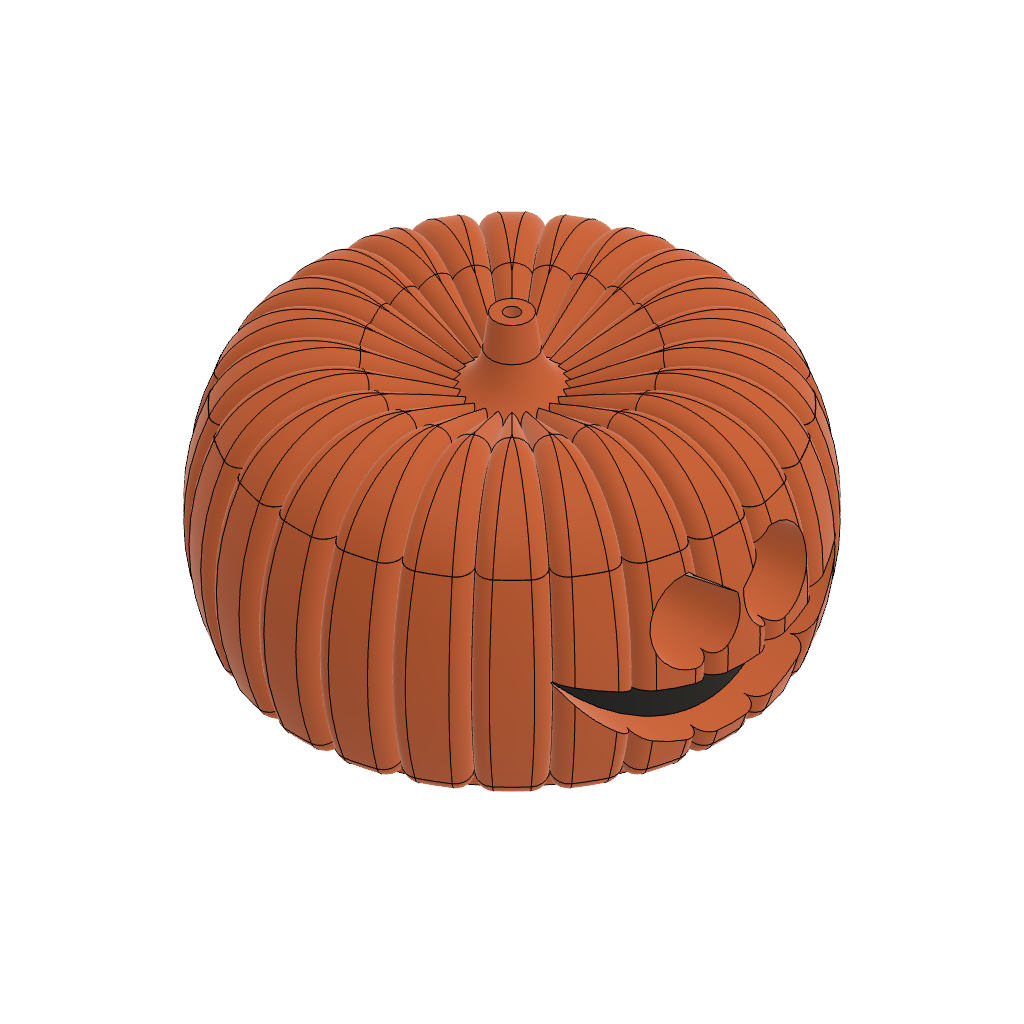
TinyEngineerHalloween (Autodesk Fusion 360 design; units mm, degrees)
part number: 2026-08-31-21-58-55-159
part number: 2026-08-31-22-02-30-810
part number: 2026-08-31-23-17-40-355
part number: 2026-08-31-23-21-15-111
part number: 2026-09-02-10-24-00-688
part number: 2026-09-25-21-20-39-307
part number: 2026-09-26-07-19-26-809
Autodesk Fusion 360 part; units mm, degrees
(part 1 of 2)
sketch "servo_profile" plane through (0, 0, 0) normal (0, 0, 1) x (1, 0, 0) in component "Servo"
  line L0 (-16.9, -13.6) -> (-16.9, -30.6) construction
  line L1 (-16.9, -30.6) -> (5.8, -30.6) construction
  line L2 (5.8, -30.6) -> (5.8, -13.6) construction
  line L3 (5.8, -13.6) -> (10.6, -13.6) construction
  line L4 (10.6, -13.6) -> (10.6, -11.2) construction
  line L5 (10.6, -11.2) -> (5.8, -11.2) construction
  line L6 (5.8, -3.3) -> (-9.1, -3.3) construction
  line L7 (-9.1, -3.3) -> (-9.1, -6.8) construction
  line L8 (-9.1, -6.8) -> (-16.9, -6.8) construction
  line L9 (-16.9, -6.8) -> (-16.9, -11.2) construction
  line L10 (-16.9, -11.2) -> (-21.7, -11.2) construction
  line L11 (-21.7, -11.2) -> (-21.7, -13.6) construction
  line L12 (-21.7, -13.6) -> (-16.9, -13.6) construction
  line L13 (0, -3.3) -> (0, 0) construction
  line L14 (5.8, -3.3) -> (5.8, -11.2) construction
  line L15 (-17.2, -10.9) -> (-22, -10.9)
  line L16 (-22, -10.9) -> (-22, -13.9)
  line L17 (-22, -13.9) -> (-17.2, -13.9)
  line L18 (-17.2, -13.9) -> (-17.2, -30.9)
  line L19 (-17.2, -30.9) -> (6.1, -30.9)
  line L20 (6.1, -30.9) -> (6.1, -13.9)
  line L21 (6.1, -13.9) -> (10.9, -13.9)
  line L22 (10.9, -13.9) -> (10.9, -10.9)
  line L23 (10.9, -10.9) -> (6.1, -10.9)
  line L24 (6.1, -3) -> (6.1, -10.9)
  line L25 (6.1, -3) -> (-9.4, -3)
  line L26 (-9.4, -3) -> (-9.4, -6.5)
  line L27 (-9.4, -6.5) -> (-17.2, -6.5)
  line L28 (-17.2, -6.5) -> (-17.2, -10.9)
  line L29 (-9.1, -3.3) -> (-16.9, -3.3) construction
  line L30 (-16.9, -3.3) -> (-16.9, -6.8) construction
  dimension "d2" = 22.7
  dimension "d6" = 17
  dimension "d7" = 2.4
  dimension "d8" = 4.8
  dimension "d13" = 4.4
  dimension "d17" = 5.8
  dimension "d20" = 3.3
  dimension "d40" = 0.3
  dimension "d115" = 3.5
  dimension "d116" = 7.8
  constraint vertical L0
  constraint perpendicular L0 L1
  constraint perpendicular L1 L2
  constraint perpendicular L0 L3
  constraint perpendicular L3 L4
  constraint perpendicular L4 L5
  constraint perpendicular L6 L7
  constraint perpendicular L7 L8
  constraint perpendicular L8 L9
  constraint perpendicular L9 L10
  constraint perpendicular L10 L11
  constraint perpendicular L0 L12
  constraint equal L0 L2
  constraint equal L4 L11
  constraint collinear L0 L9
  constraint equal L3 L12
  constraint coincident L6 L13.start
  constraint perpendicular L6 L13
  constraint coincident L13.end origin
  constraint perpendicular L5 L14
  constraint collinear L2 L14
  constraint coincident L6.start L14.start
  constraint perpendicular L26 L29
  constraint perpendicular L29 L30
  measures "d2" distance of L0.end L1.end
  measures "d6" distance of L0.start L0.end
  measures "d7" distance of L10.end L11.end
  measures "d8" distance of L2.end L3.end
  measures "d13" distance of L8.end L9.end
  measures "d17" distance of L13 L14
  measures "d20" distance of L13.start L13.end
  measures "d115" distance of L8.end L29.end
  measures "d116" distance of L6.end L29.end
extrude "Extrude1" add sketch "servo_profile" along normal mid plane 12.8 makes body 1 in component "Servo"
sketch "shaft" plane through (0, -3, 0) normal (0, 1, 0) x (-1, 0, 0) in component "Servo"
  line L0 (9, -5.75) -> (9, 5.75)
  line L1 (9, 5.75) -> (-3, 5.75)
  line L2 (-3, 5.75) -> (-3, -5.75)
  line L3 (-3, -5.75) -> (9, -5.75)
  circle A0 centre (0, 0) radius 2.7
  line L4 (9.4, -6.4) -> (9.4, 6.4)
  line L5 (9.4, 6.4) -> (-6.1, 6.4)
  line L6 (-6.1, 6.4) -> (-6.1, -6.4)
  line L7 (-6.1, -6.4) -> (9.4, -6.4)
  dimension "d25" = 5.4
  constraint coincident A0.centre origin
  measures "d25" diameter of A0
extrude "Extrude2" add sketch "shaft" along normal blind 3.6 contours A0 bodies 1 in component "Servo"
sketch "mount" plane through (0, -3, 0) normal (0, 1, 0) x (-1, 0, 0) in component "Servo"
  circle A0 centre (-8.27, 0) radius 1.4
  circle A1 centre (19.37, 0) radius 1.4
  line L0 (19.37, 0) -> (-8.27, 0) construction
  line L1 (0, 0) -> (-5.8, 0) construction
  line L2 (-5.8, 0) -> (-10.6, 0) construction
  line L3 (-10.6, 0) -> (-10.6, -6.1) construction
  line L4 (-10.6, -6.1) -> (-8.27, -6.1) construction
  line L5 (-8.27, -6.1) -> (-8.27, 0) construction
  dimension "d31" = 2.8
  dimension "d32" = 5.8
  dimension "d33" = 4.8
  dimension "d34" = 6.1
  dimension "d35" = 2.33
  dimension "d36" = 6.1
  dimension "d37" = 19.37
  constraint coincident A1.centre L0.start
  constraint coincident A0.centre L0.end
  constraint horizontal L0
  constraint equal A0 A1
  constraint coincident L1.start origin
  constraint horizontal L1
  constraint parallel L1 L2
  constraint perpendicular L2 L3
  constraint perpendicular L3 L4
  constraint vertical L5
  measures "d31" diameter of A0
  measures "d32" distance of L1.start L1.end
  measures "d33" distance of L1.end L2.end
  measures "d34" distance of L2.end L3.end
  measures "d35" distance of L3.end L4.end
  measures "d36" distance of A0.centre L4.end
  measures "d37" distance of L1.start A1.centre
extrude "Extrude3" cut sketch "mount" against normal through all bodies 1 in component "Servo"
sketch "Sketch1" plane through (0, 0, 0) normal (0, 0, 1) x (1, 0, 0) in component "OLED"
  line L0 (-4.7, -18.25) -> (0, -18.25)
  line L1 (0, -18.25) -> (0, 18.25)
  line L2 (0, 18.25) -> (-8.7, 18.25)
  line L3 (-8.7, 18.25) -> (-8.7, 10.25)
  line L4 (-8.7, 10.25) -> (-4.7, 10.25)
  line L5 (-4.7, 10.25) -> (-4.7, -18.25)
  dimension "d195" = 36.5
  dimension "d196" = 4.7
  dimension "d197" = 8.7
  dimension "d202" = 8
  constraint horizontal L0
  constraint perpendicular L0 L1
  constraint perpendicular L1 L2
  constraint perpendicular L2 L3
  constraint perpendicular L3 L4
  constraint perpendicular L4 L5
  constraint midpoint origin L1
  measures "d195" distance of L0.end L1.end
  measures "d196" distance of L0.start L0.end
  measures "d197" distance of L1.end L2.end
  measures "d202" distance of L2.end L3.end
extrude "Extrude1'" add sketch "Sketch1" along normal blind 12.5 separate body makes body 2 in component "OLED"
sketch "servo_case" plane through (0, 0, -6.4) normal (0, 0, -1) x (1, 0, 0) in component "Head"
  line L0 (-9.4, 3) -> (6.1, 3)
  line L1 (6.1, 3) -> (6.1, 10.9)
  line L2 (6.1, 10.9) -> (10.9, 10.9)
  line L3 (10.9, 13.9) -> (6.1, 13.9)
  line L4 (6.1, 13.9) -> (6.1, 30.9)
  line L5 (6.1, 30.9) -> (-17.2, 30.9)
  line L6 (-17.2, 30.9) -> (-17.2, 13.9)
  line L7 (-17.2, 13.9) -> (-22, 13.9)
  line L8 (-22, 10.9) -> (-17.2, 10.9)
  line L9 (-17.2, 10.9) -> (-17.2, 6.5)
  line L10 (-17.2, 6.5) -> (-9.4, 6.5)
  line L11 (-9.4, 6.5) -> (-9.4, 3)
  line L12 (12.1, 3) -> (-23.5, 3)
  line L13 (-23.5, 3) -> (-23.5, 35.9) construction
  line L14 (-23.5, 35.9) -> (12.1, 35.9)
  line L15 (12.1, 35.9) -> (12.1, 3)
  line L16 (6.1, 3) -> (6.1, 10.9)
  line L17 (6.1, 10.9) -> (10.9, 10.9)
  line L18 (10.9, 10.9) -> (10.9, 13.9)
  line L19 (10.9, 13.9) -> (6.1, 13.9)
  line L20 (6.1, 13.9) -> (6.1, 30.9)
  line L21 (6.1, 30.9) -> (-17.2, 30.9)
  line L22 (-17.2, 30.9) -> (-17.2, 13.9)
  line L23 (-17.2, 13.9) -> (-22, 13.9)
  line L24 (-22, 13.9) -> (-22, 10.9)
  line L25 (-22, 10.9) -> (-17.2, 10.9)
  line L26 (-17.2, 10.9) -> (-17.2, 6.5)
  line L27 (-17.2, 6.5) -> (-9.4, 6.5)
  line L28 (-9.4, 6.5) -> (-9.4, 3)
  line L29 (12.1, 35.9) -> (12.1, 24.9)
  line L30 (12.1, 24.9) -> (11.6, 24.9) construction
  line L31 (8.6, 34.4) -> (8.6, 32.9) construction
  line L32 (7.1, 32.9) -> (6.1, 32.9)
  line L33 (4.1, 32.9) -> (4.1, 30.9) construction
  line L34 (11.6, 24.9) -> (11.6, 35.9)
  line L35 (11.6, 24.9) -> (6.1, 24.9)
  line L36 (-5.55, 30.9) -> (-5.55, 19) construction
  circle A0 centre (-5.55, 19) radius 9.85
  line L37 (10.9, 10.9) -> (10.9, 13.9)
  line L38 (-22, 13.9) -> (-22, 10.9)
  line L39 (8.6, 34.4) -> (7.1, 34.4) construction
  line L40 (8.6, 35.9) -> (8.6, 34.4) construction
  arc A1 (7.1, 32.9) -> (7.1, 35.9) centre (7.1, 34.4) ccw
  line L41 (8.6, 32.9) -> (7.1, 32.9) construction
  arc A2 (6.1, 32.9) -> (4.1, 30.9) centre (6.1, 30.9) ccw
  line L42 (6.1, 32.9) -> (4.1, 32.9) construction
  line L43 (-53.5, 3) -> (-53.5, 35.9) construction
  line L44 (-53.5, 3) -> (-23.5, 3) construction
  line L45 (12.1, 19.45) -> (0.3, 19.45) construction
  circle A3 centre (0.3, 19.45) radius 28.9317
  line L46 (12.1, 3) -> (12.1, -6.966)
  line L47 (12.1, 35.9) -> (12.1, 45.866)
  line L48 (-21.2, 35.9) -> (-21.2, 38.8096)
  line L49 (-21.2, 3) -> (-21.2, 0.0904)
  line L50 (-16.6452, 35.9) -> (-16.6452, 42.9)
  line L51 (-16.6452, 3) -> (-16.6452, -4)
  line L52 (-17.2, 16.9) -> (-28.5191, 16.9)
  line L53 (-17.2, 27.9) -> (-27.3702, 27.9)
  point P0 (8.6, 34.4)
  dimension "d42" = 5
  dimension "d61" = 8
  dimension "d62" = 2
  dimension "d71" = 0.5
  dimension "d72" = 3
  dimension "d74" = 2
  dimension "d82" = 11.9
  dimension "d83" = 19.7
  dimension "d89" = 6.3
  dimension "d90" = 6
  dimension "head_width" = 32.9
  dimension "d267" = 30
  dimension "d1884" = 5.8
  dimension "d1981" = 2.3
  dimension "d1982" = 7
  dimension "d1999" = 3
  dimension "d2000" = 3
  dimension "d2054" = 57.8634
  constraint horizontal L12
  constraint vertical L13
  constraint horizontal L14
  constraint vertical L15
  constraint collinear L0 L12
  constraint coincident L0.end L1.start
  constraint coincident L1.end L2.start
  constraint coincident L2.end L17.end
  constraint coincident L3.start L18.end
  constraint coincident L3.end L4.start
  constraint coincident L4.end L5.start
  constraint coincident L5.end L6.start
  constraint coincident L6.end L7.start
  constraint coincident L7.end L23.end
  constraint coincident L8.start L24.end
  constraint coincident L8.end L9.start
  constraint coincident L9.end L10.start
  constraint coincident L10.end L11.start
  constraint coincident L0.start L11.end
  constraint coincident L15 L29.end
  constraint coincident L20 L35.end
  constraint perpendicular L20 L30
  constraint coincident L14 L40.start
  constraint perpendicular L14 L31
  constraint perpendicular L31 L32
  constraint coincident L21 L33.end
  constraint perpendicular L21 L33
  constraint coincident L14 L34.end
  constraint perpendicular L14 L34
  constraint perpendicular L20 L35
  constraint midpoint L21 L36.start
  constraint perpendicular L21 L36
  constraint coincident L36.end A0.centre
  constraint perpendicular L31 L39
  constraint perpendicular L14 L40
  constraint coincident P0 L31.start
  constraint equal L39 L40
  constraint equal L31 L40
  constraint coincident L14 A1.end
  constraint coincident L39.end A1.centre
  constraint perpendicular L31 L41
  constraint perpendicular L31 L42
  constraint tangent L14 A1
  constraint perpendicular L21 L43
  constraint perpendicular L43 L44
  constraint midpoint L15 L45.start
  constraint perpendicular L20 L45
  constraint coincident L45.end A3.centre
  constraint coincident L12.end A3
  constraint coincident A3 L46.end
  constraint perpendicular L12 L46
  constraint coincident A3 L47.end
  constraint perpendicular L14 L47
  constraint coincident L14 L48.start
  constraint coincident A3 L48.end
  constraint perpendicular L14 L48
  constraint coincident L12 L49.start
  constraint coincident A3 L49.end
  constraint perpendicular L12 L49
  constraint collinear L48 L49
  constraint coincident L14 L50.start
  constraint coincident A3 L50.end
  constraint perpendicular L14 L50
  constraint coincident L12 L51.start
  constraint coincident A3 L51.end
  constraint perpendicular L12 L51
  constraint collinear L50 L51
  constraint coincident L22 L52.start
  constraint coincident A3 L52.end
  constraint perpendicular L13 L52
  constraint coincident L22 L53.start
  constraint coincident A3 L53.end
  constraint perpendicular L13 L53
  measures "d42" distance of L5 L14
  measures "d61" distance of L30 L32
  measures "d62" distance of L33.start L33.end
  measures "d71" distance of L29 L34
  measures "d72" distance of L40.start L34
  measures "d74" distance of L4.end L33
  measures "d82" distance of L36.start L36.end
  measures "d83" diameter of A0
  measures "d89" distance of L13 L26
  measures "d90" distance of L15 L16
  measures "head_width" distance of L43.start L43.end
  measures "d267" distance of L12.end L43.start
  measures "d1884" horizontal distance of L0.end L45.end
  measures "d1981" distance of L13.end L48.start
  measures "d1982" distance of L50.start L50.end
  measures "d1999" distance of L5.end L53.start
  measures "d2000" distance of L23 L52
  measures "d2054" diameter of A3
extrude "Extrude1''" add sketch "servo_case" along normal blind 1.8 separate body contours L0 L1 L2 L3 L4 L5 L6 L7 L8 L9 L10 L11 L12 L16 L17 L18 L19 L20 L21 L22 L23 L24 L25 L26 L27 L28 L37 L38 | L6 L7 L8 L9 L10 L11 L12 L22 L23 L24 L25 L26 L27 L28 L38 A3 L52 | L1 L2 L3 L4 L12 L14 L15 L16 L17 L18 L19 L20 L29 L34 L35 L37 | L12 A3 L49 L51 | L15 L29 A3 L46 L47 | L6 L22 A3 L52 L53 | L4 L5 L14 L20 L21 L32 L34 L35 A1 A2 | L5 L6 L14 L21 L22 L32 A1 A2 A3 L53 | L14 A3 L48 L50 makes body 3 in component "Head"
fillet "Fillet8" radius 5 2 edges at (-16.6452, -35.9, -7.3) (-16.6452, -3, -7.3) on bodies 3 in component "Head"
fillet "Fillet8" radius 1 2 edges at (-16.6452, -42.9, -7.3) (-16.6452, 4, -7.3) on bodies 3 in component "Head"
extrude "Extrude2'" add sketch "servo_case" against normal blind 12.8 contours L6 L7 L8 L9 L10 L11 L12 L22 L23 L24 L25 L26 L27 L28 L38 A3 L52 | L1 L2 L3 L4 L12 L14 L15 L16 L17 L18 L19 L20 L29 L34 L35 L37 | L6 L22 A3 L52 L53 | L5 L6 L14 L21 L22 L32 A1 A2 A3 L53 bodies 3 in component "Head"
extrude "Extrude19" add 1 faces at (17.8106, -19.45, -6.4) along direction (0, 0, 1) up to surface (12.8 mm away) separate body on bodies 3 makes body 4 in component "Head"
fillet "Fillet12" radius 2 4 edges at (12.1, 6.966, -7.3) (12.1, -45.866, -7.3) (12.1, 6.966, 0) (12.1, -45.866, 0) on bodies 3 4 in component "Head"
shell "Shell1" thickness 1.5 removed faces 1 at (17.8106, -19.45, 6.4) on bodies 4 in component "Head"
combine "Combine1" operation add target body 3 tool bodies 4 in component "Head"
extrude "Extrude14" add sketch "servo_case" against normal blind 1 contours L4 L5 L14 L20 L21 L32 L34 L35 A1 A2 bodies 3 in component "Head"
fillet "Fillet6" radius 2 1 edges at (11.6, -24.9, 0) on bodies 3 in component "Head"
sketch "axis_mount" plane through (0, -35.9, 0) normal (0, -1, 0) x (1, 0, 0) in component "Head"
  line L0 (12.1, 6.4) -> (11.6, 6.4)
  circle A0 centre (0, 0) radius 2.7 construction
  circle A1 centre (0, 0) radius 1.2
  line L1 (11.6, 6.4) -> (11.6, -5.4)
  line L2 (11.6, -5.4) -> (7.1, -5.4)
  line L3 (-23.5, 6.4) -> (-23.5, -8.2)
  line L4 (-23.5, -8.2) -> (-21.2, -8.2)
  line L5 (7.1, -5.4) -> (7.1, 6.4)
  line L6 (7.1, 6.4) -> (-23.5, 6.4)
  line L7 (-21.2, -8.2) -> (-21.2, -6.4)
  line L8 (-21.2, -6.4) -> (-11.6452, -6.4)
  line L9 (-11.6452, -6.4) -> (-11.6452, -8.2)
  line L10 (-11.6452, -8.2) -> (12.1, -8.2)
  line L11 (12.1, -8.2) -> (12.1, 6.4)
  dimension "d106" = 2.4
  constraint concentric A0 A1
  measures "d106" diameter of A1
extrude "Extrude6" cut sketch "axis_mount" against normal up to surface (5 mm away) contours A1 bodies 3 in component "Head"
ref_plane "WorkPlane2" through (-28.6317, -19.45, -3.5582) normal (-1, 0, 0) x (0, -1, 0) in component "Head"
sketch "mount_hole" plane through (-28.6317, 0, 0) normal (-1, 0, 0) x (0, -1, 0) in component "Head"
  line L0 (3, -8.2) -> (35.9, -8.2)
  line L1 (19.45, -8.2) -> (19.45, -4.55)
  circle A0 centre (19.45, -4.55) radius 1.05
  dimension "d2018" = 3.65
  dimension "d2019" = 2.1
  constraint midpoint L0 L1.start
  constraint perpendicular L0 L1
  constraint coincident L1.end A0.centre
  measures "d2018" distance of L1.start L1.end
  measures "d2019" diameter of A0
extrude "Extrude15" cut sketch "mount_hole" against normal up to surface (9.9317 mm away) bodies 3 in component "Head"
extrude "Extrude16" cut sketch "servo_case" along normal up to surface (8.6 mm away) from surface at -12.8 contours L6 L22 A3 L52 L53 bodies 3 in component "Head"
fillet "Fillet11" radius 3 2 edges at (-28.5191, -16.9, 2.1) (-27.3702, -27.9, 2.1) on bodies 3 in component "Head"
sketch "Sketch8" plane through (0, -3, 0) normal (0, 1, 0) x (-1, 0, 0) in component "Head"
  line L0 (11.6452, -8.2) -> (11.6452, -6.4)
  line L1 (11.6452, -6.4) -> (21.2, -6.4)
  line L2 (21.2, -6.4) -> (21.2, -8.2)
  line L3 (21.2, -8.2) -> (23.5, -8.2)
  line L4 (23.5, -8.2) -> (23.5, 6.4)
  line L5 (23.5, 6.4) -> (9.4, 6.4)
  line L6 (9.4, 6.4) -> (9.4, -6.4)
  line L7 (9.4, -6.4) -> (-6.1, -6.4)
  line L8 (-6.1, -6.4) -> (-6.1, 6.4)
  line L9 (-6.1, 6.4) -> (-12.1, 6.4)
  line L10 (-12.1, 6.4) -> (-12.1, -8.2)
  line L11 (-12.1, -8.2) -> (11.6452, -8.2)
  circle A0 centre (-8.27, 0) radius 1.4 construction
  circle A1 centre (19.37, 0) radius 1.4 construction
  circle A2 centre (-8.27, 0) radius 1.05
  circle A3 centre (19.37, 0) radius 1.05
  circle A4 centre (-8.27, 0) radius 2
  circle A5 centre (19.37, 0) radius 2
  dimension "d2027" = 2.1
  dimension "d2028" = 4
  constraint concentric A0 A2
  constraint concentric A1 A3
  constraint equal A2 A3
  constraint concentric A2 A4
  constraint concentric A3 A5
  constraint equal A4 A5
  measures "d2027" diameter of A2
  measures "d2028" diameter of A5
extrude "Extrude17" cut sketch "Sketch8" against normal up to surface (27.9 mm away) contours A2 | A3 bodies 3 in component "Head"
extrude "Extrude18" cut sketch "Sketch8" against normal blind 2 contours A4 | A5 bodies 3 in component "Head"
sketch "base" plane through (0, 0, -8.2) normal (0, 0, -1) x (1, 0, 0) in component "Cover"
  circle A0 centre (-5.55, 19) radius 9.85
  arc A1 (-18.2875, 41.6209) -> (-21.2, 38.8096) centre (0.3, 19.45) ccw
  line L0 (-23.5, 3) -> (-21.2, 3)
  line L1 (12.1, 3) -> (12.1, -3.6774)
  arc A2 (15.1248, -5.3949) -> (15.1248, 44.2949) centre (0.3, 19.45) ccw
  line L2 (12.1, 42.5774) -> (12.1, 35.9)
  line L3 (12.1, 35.9) -> (-11.6452, 35.9)
  line L4 (-19.793, 40.2662) -> (0.3, 19.45) construction
  line L5 (6.1, 10.9) -> (6.1, 3)
  circle A3 centre (0.3, 19.45) radius 29.2317
  circle A4 centre (0.3, 19.45) radius 29.6317
  line L6 (-19.793, 40.2662) -> (-20.0013, 40.4821) construction
  line L7 (-20.0013, 40.4821) -> (-20.2791, 40.7699) construction
  line L8 (-21.6568, 38.7474) -> (-21.6568, 36.2)
  line L9 (-21.6568, 36.2) -> (-23.6568, 36.2)
  line L10 (-21.8636, 38.5096) -> (-21.6568, 38.5096)
  line L11 (-21.6568, 0.1526) -> (-21.6568, 38.5096)
  arc A5 (-16.6451, 40.8621) -> (-11.6452, 35.9) centre (-11.6452, 40.9) ccw
  line L12 (-21.2, 38.8096) -> (-21.2, 35.9)
  line L13 (-21.2, 35.9) -> (-23.5, 35.9)
  line L14 (-21.2, 3) -> (-21.2, 0.0904)
  arc A6 (-21.2, 0.0904) -> (-18.2875, -2.7209) centre (0.3, 19.45) ccw
  arc A7 (-11.6452, 3) -> (-16.6451, -1.9621) centre (-11.6452, -2) ccw
  line L15 (-11.6452, 3) -> (12.1, 3)
  line L16 (-21.6568, 2.7) -> (-23.6568, 2.7)
  arc A8 (-18.2875, -2.7209) -> (-16.6451, -1.9621) centre (-17.645, -1.9546) ccw
  arc A9 (-16.6451, 40.8621) -> (-18.2875, 41.6209) centre (-17.645, 40.8546) ccw
  arc A10 (15.1248, 44.2949) -> (12.1, 42.5774) centre (14.1, 42.5774) ccw
  arc A11 (12.1, -3.6774) -> (15.1248, -5.3949) centre (14.1, -3.6774) ccw
  arc A12 (-23.5, 35.9) -> (-23.5, 3) centre (0.3, 19.45) ccw
  dimension "d1885" = 5.8
  dimension "d1886" = 0.3
  dimension "d1887" = 0.4
  dimension "d1890" = 0.3
  dimension "d1891" = 0.3
  dimension "d1892" = 2
  dimension "d1985" = 2
  constraint midpoint A1 L4.start
  constraint perpendicular A1 L4
  constraint concentric A1 A3
  constraint coincident A1.centre A2.centre
  constraint coincident A3 L6.end
  constraint perpendicular A3 L6
  constraint coincident A4 L7.end
  constraint perpendicular A4 L7
  constraint coincident A3 L8.start
  constraint perpendicular L3 L8
  constraint coincident A3 L9.end
  constraint perpendicular L8 L9
  constraint coincident A3 L10.start
  constraint parallel L3 L10
  constraint coincident A3 L11.start
  constraint perpendicular L10 L11
  constraint collinear L8 L11
  constraint coincident L11 L16.start
  constraint coincident A3 L16.end
  constraint perpendicular L11 L16
  measures "d1885" horizontal distance of A1.centre L5.end
  measures "d1886" distance of L4.start L6.end
  measures "d1887" distance of L6.end L7.end
  measures "d1890" vertical distance of L3.end L8.end
  measures "d1891" vertical distance of A1.end L10.end
  measures "d1892" distance of L8.end L9.end
  measures "d1985" distance of L16.start L16.end
extrude "Extrude1'''" add sketch "base" against normal up to surface (14.6 mm away) separate body contours A3 L8 L9 L10 L11 | A3 L11 L16 | A3 L8 L10 | A4 makes body 5 in component "Cover"
sketch "oled_profile" plane through (0, 0, 6.4) normal (0, 0, 1) x (-1, 0, 0) in component "Cover"
  arc A0 (21.6568, 38.7474) -> (21.6568, 0.1526) centre (-0.3, 19.45) ccw
  line L0 (21.6568, 38.7474) -> (21.6568, 36.2)
  circle A1 centre (-0.3, 19.45) radius 29.6317
  line L1 (-22.8918, 38) -> (-17.5918, 38)
  line L2 (-17.5918, 9.5) -> (-13.5918, 9.5)
  line L3 (-17.5918, 9.5) -> (-17.5918, 38)
  line L4 (-13.5918, 9.5) -> (-13.5918, 0.9)
  line L5 (-13.5918, 0.9) -> (-22.8918, 0.9)
  line L6 (-22.8918, 0.9) -> (-22.8918, 38)
  line L7 (-19.9918, 0.9) -> (-19.9918, -2.1538)
  line L8 (-13.5918, 0.9) -> (-13.5918, -4.585)
  line L9 (-13.5918, -4.585) -> (-13.5918, -6.585) construction
  line L10 (-13.5918, -4.585) -> (-12.0918, -4.585)
  line L11 (-12.0918, -4.585) -> (-12.0918, 46.1978)
  arc A2 (-12.0918, 46.1978) -> (-19.9918, -2.1538) centre (-0.3, 19.45) ccw
  line L12 (21.6568, 36.2) -> (23.6568, 36.2)
  line L13 (21.6568, 2.7) -> (21.6568, 0.1526)
  arc A3 (23.6568, 2.7) -> (23.6568, 36.2) centre (-0.3, 19.45) ccw
  line L14 (23.6568, 2.7) -> (21.6568, 2.7)
  line L15 (-17.5918, 9.5) -> (-22.8918, 9.5)
  line L16 (-17.5918, 33) -> (-22.8918, 33)
  line L17 (21.6568, 36.2) -> (21.6568, 2.7)
  dimension "d1895" = 37.1
  dimension "d1896" = 5.3
  dimension "d1897" = 8.6
  dimension "d1898" = 9.3
  dimension "d1962" = 2.9
  dimension "d1963" = 2
  dimension "d1964" = 1.5
  dimension "d1997" = 5
  constraint horizontal L1
  constraint parallel L1 L2
  constraint perpendicular L1 L3
  constraint perpendicular L2 L4
  constraint perpendicular L4 L5
  constraint perpendicular L5 L6
  constraint coincident A0 L1.start
  constraint coincident A0 L5.end
  constraint coincident L5 L7.start
  constraint coincident A0 L7.end
  constraint perpendicular L5 L7
  constraint perpendicular L5 L8
  constraint coincident A0 L9.end
  constraint parallel L8 L9
  constraint perpendicular L9 L10
  constraint coincident A0 L11.end
  constraint vertical L11
  constraint coincident A0.centre A1.centre
  constraint coincident L6 L15.end
  constraint perpendicular L6 L15
  constraint coincident L3 L16.start
  constraint coincident L6 L16.end
  constraint perpendicular L6 L16
  constraint coincident L0.end L12.start
  constraint coincident L13.start L14.end
  measures "d1895" distance of L1.start L5.end
  measures "d1896" distance of L1.start L1.end
  measures "d1897" distance of L2.end L4.end
  measures "d1898" distance of L4.end L5.end
  measures "d1962" horizontal distance of L5.end L7.end
  measures "d1963" distance of L8.end L9.end
  measures "d1964" distance of L8.end L10.end
  measures "d1997" distance of L1.end L16.start
extrude "Extrude2''" add sketch "oled_profile" along normal blind 13.1 contours A0 L1 L2 L3 L4 L8 L10 L11 A2 | L12 A3 L14 L17 | A0 L6 A2 | A0 L5 L7 A2 | A1 bodies 5 in component "Cover"
sketch "roof" plane through (0, 0, 19.5) normal (0, 0, 1) x (-1, 0, 0) in component "Cover"
  circle A0 centre (-0.3, 19.45) radius 29.6317
  line L0 (-19.9918, 0.9) -> (-22.8918, 0.9)
  line L1 (-13.5918, -4.585) -> (-12.0918, -4.585)
  line L2 (-12.0918, -4.585) -> (-12.0918, 46.1978)
  arc A1 (21.6568, 38.7474) -> (-12.0918, 46.1978) centre (-0.3, 19.45) ccw
  line L3 (-19.9918, -2.1538) -> (-19.9918, 0.9)
  line L4 (21.6568, 38.7474) -> (21.6568, 0.1526)
  line L5 (-22.8918, 0.9) -> (-22.8918, 38)
  line L6 (-22.8918, 38) -> (-17.5918, 38)
  line L7 (-17.5918, 38) -> (-17.5918, 9.5)
  line L8 (-17.5918, 9.5) -> (-13.5918, 9.5)
  line L9 (-13.5918, 9.5) -> (-13.5918, -4.585)
  arc A2 (-19.9918, -2.1538) -> (21.6568, 0.1526) centre (-0.3, 19.45) ccw
extrude "Extrude3'" add sketch "oled_profile" along normal blind 1.5 from surface at 13.1 contours A0 L0 L5 L7 L8 L10 L11 L13 L17 | A0 L1 L2 L3 L4 L8 L10 L11 A2 | L12 A3 L14 L17 | A0 L6 A2 | L1 L3 L6 L16 | A0 L5 L7 A2 | L2 L4 L5 L6 L15 | A1 bodies 5 in component "Cover"
ref_plane "WorkPlane1" through (0.3, 10.1817, 1.8046) normal (0, 1, 0) x (1, 0, 0) in component "Cover"
ref_plane "WorkPlane2" through (0.3, -49.0817, 2.5448) normal (0, -1, 0) x (-1, 0, 0) in component "Cover"
ref_plane "WorkPlane3" through (0.3, -19.45, 1.8046) normal (0, 1, 0) x (1, 0, 0) in component "Cover"
sketch "pumpkin_surface" plane through (0, -19.45, 0) normal (0, 1, 0) x (1, 0, 0) in component "Cover"
  line L0 (29.9317, 8.2) -> (-29.3317, 8.2)
  line L1 (-29.3317, -21) -> (-29.3317, 8.2)
  line L2 (-29.3317, 4.2) -> (-29.3317, 8.2) construction
  line L3 (-29.3317, 4.2) -> (-32.3317, 6.2002) construction
  line L4 (-29.3317, -21) -> (-32.3317, -21)
  line L5 (-32.3317, -21) -> (-32.3317, 6.2002) construction
  line L6 (-32.3317, -7.3999) -> (0.3, -7.3999) construction
  arc A0 (-32.3317, 6.2002) -> (-32.3317, -21) centre (0.3, -7.3999) ccw
  arc A1 (-29.3317, 8.2) -> (-32.3317, 6.2002) centre (-29.3317, 4.9499) ccw
  line L7 (-29.3317, -21) -> (29.9317, -21)
  line L8 (0.3, -21) -> (0.3, 8.2) construction
  dimension "d1928" = 4
  dimension "d1946" = 3
  constraint coincident L0.end L1.end
  constraint coincident L1 L2.start
  constraint midpoint L5 L6.start
  constraint perpendicular L5 L6
  constraint coincident L6.end A0.centre
  constraint vertical L5
  constraint tangent A0 A1
  constraint tangent L0 A1
  constraint coincident L4.end L5.start
  constraint horizontal L4
  constraint coincident L1.start L4.start
  constraint midpoint L7 L8.start
  constraint midpoint L0 L8.end
  constraint coincident L6.end L8
  measures "d1928" distance of L2.start L0.end
  measures "d1946" distance of L1.start L4.end
revolve "Revolve1" add sketch "pumpkin_surface" angle 7.5 about axis through (0.3, -19.45, 21) along (0, 0, -1) second angle 7.5 separate body makes body 6 in component "Cover"
fillet "Fillet1" radius 2.0665 4 edges at (-34.7499, -24.0644, 7.3999) (-30.8655, -23.553, -7.6542) (-34.7499, -14.8356, 7.3999) (-30.8655, -15.347, -7.6542) on bodies 6 in component "Cover"
pattern_circular "C-Pattern1" count 24 over 360 about axis through (0.3, -19.45, 21) along (0, 0, -1) of bodies 6 makes body 7 at (-28.3734, -11.9752, 11.2667) makes body 8 at (-25.4618, -4.8087, 11.2667) makes body 9 at (-20.7945, 1.36, 11.2667) makes body 10 at (-14.6897, 6.1106, 11.2667) makes body 11 at (-7.5634, 9.1193, 11.2667) makes body 12 at (0.0988, 10.181, 11.2667) makes body 13 at (7.7748, 9.2234, 11.2667) makes body 14 at (14.9413, 6.3118, 11.2667) makes body 15 at (21.11, 1.6445, 11.2667) makes body 16 at (25.8606, -4.4603, 11.2667) makes body 17 at (28.8693, -11.5866, 11.2667) makes body 18 at (29.931, -19.2488, 11.2667) makes body 19 at (28.9734, -26.9248, 11.2667) makes body 20 at (26.0618, -34.0913, 11.2667) makes body 21 at (21.3945, -40.26, 11.2667) makes body 22 at (15.2897, -45.0106, 11.2667) makes body 23 at (8.1634, -48.0193, 11.2667) makes body 24 at (0.5012, -49.081, 11.2667) makes body 25 at (-7.1748, -48.1234, 11.2667) makes body 26 at (-14.3413, -45.2118, 11.2667) makes body 27 at (-20.51, -40.5445, 11.2667) makes body 28 at (-25.2606, -34.4397, 11.2667) makes body 29 at (-28.2693, -27.3134, 11.2667) in component "Cover"
combine "Combine1'" operation add target body 5 tool bodies 18 22 9 12 14 13 15 16 11 10 17 7 25 28 26 29 6 8 27 24 23 21 19 20 in component "Cover"
sketch "face" plane through (22.8918, 0, 0) normal (-1, 0, 0) x (0, -1, 0) in component "Cover"
  line L0 (38, 19.5) -> (33, 19.5)
  line L1 (33, 19.5) -> (33, 21)
  line L2 (33, 21) -> (9.5, 21)
  line L3 (9.5, 21) -> (9.5, 19.5)
  line L4 (9.45, 19.5) -> (29.45, 19.5) construction
  line L5 (29.45, 19.5) -> (29.45, 6.4) construction
  line L6 (29.45, 6.4) -> (9.45, 6.4) construction
  line L7 (9.45, 6.4) -> (9.45, 19.5) construction
  line L8 (38, 6.4) -> (29.45, 6.4) construction
  line L9 (9.45, 6.4) -> (0.9, 6.4) construction
  line L10 (16.95, 19.5) -> (16.95, 6.4) construction
  line L11 (21.95, 19.5) -> (21.95, 6.4) construction
  line L12 (21.95, 12.95) -> (29.45, 12.95) construction
  line L13 (16.95, 12.95) -> (9.45, 12.95) construction
  circle A0 centre (13.2, 12.95) radius 3.75
  circle A1 centre (25.7, 12.95) radius 3.75
  line L14 (16.95, 12.95) -> (9.45, 19.5)
  line L15 (21.95, 12.95) -> (29.45, 19.5)
  line L16 (36.2, -8.2) -> (2.7, -8.2)
  arc A2 (0.9, 6.4) -> (38, 6.4) centre (19.45, 47.4128) ccw
  arc A3 (0.9, 6.4) -> (38, 6.4) centre (19.45, 22.106) ccw
  line L17 (19.45, 6.4) -> (19.45, 2.4) construction
  line L18 (19.45, -2.2) -> (19.45, -8.2) construction
  line L19 (0.9, 6.4) -> (38, 6.4)
  line L20 (38, 6.4) -> (38, 19.5)
  line L21 (9.5, 19.5) -> (0.9, 19.5)
  line L22 (0.9, 19.5) -> (0.9, 6.4)
  line L23 (9.45, 12.95) -> (0.9, 12.95) construction
  dimension "d2003" = 20
  dimension "d2004" = 5
  dimension "d2055" = 6
  dimension "d2057" = 4
  constraint horizontal L4
  constraint vertical L5
  constraint horizontal L6
  constraint vertical L7
  constraint equal L8 L9
  constraint coincident L4 L10.start
  constraint coincident L6 L10.end
  constraint coincident L4 L11.start
  constraint coincident L6 L11.end
  constraint vertical L11
  constraint vertical L10
  constraint midpoint L11 L12.start
  constraint midpoint L5 L12.end
  constraint midpoint L10 L13.start
  constraint midpoint L7 L13.end
  constraint equal L12 L13
  constraint midpoint L13 A0.centre
  constraint coincident L13.start A0
  constraint midpoint L12 A1.centre
  constraint coincident L12.start A1
  constraint midpoint A2 L17.end
  constraint midpoint A3 L18.start
  constraint midpoint L16 L18.end
  constraint midpoint L22 L23.end
  constraint perpendicular L22 L23
  constraint coincident L8.start A2.end
  constraint coincident L9.end A2.start
  constraint collinear L0 L4
  constraint perpendicular L17 L19
  constraint midpoint L6 L17.start
  measures "d2003" distance of L5.end L6.end
  measures "d2004" distance of L10.start L11.start
  measures "d2055" distance of L18.start L18.end
  measures "d2057" distance of L17.start L17.end
extrude "Extrude8" cut sketch "face" against normal blind 50 draft 10 contours A2 A3 | A0 L14 | A1 L15 picked at (12.9195, 13.3482) picked at (26.6275, 13.5859) bodies 5 in component "Cover"
sketch "top_mount" plane through (0, 0, 21) normal (0, 0, 1) x (-1, 0, 0) in component "Cover"
  circle A0 centre (-0.3, 19.45) radius 1.05
  spline S0 degree 3 poles (-27.466, 37.5286) (-27.4417, 37.5651) (-27.4167, 37.6) (-27.3913, 37.6331) (-27.2402, 37.83) (-27.014, 38.0238) (-26.5708, 38.27) (-26.274, 38.3615) (-25.7453, 38.4178) (-25.4193, 38.3869) (-24.8811, 38.2326) (-24.5744, 38.0764) (-24.3468, 37.9017) knots -0.012509 -0.012509 -0.012509 -0.012509 0 0 0 0.074471 0.074471 0.152103 0.152103 0.233978 0.233978 0.320047 0.320047 0.320047 0.320047
  arc A1 (-27.466, 37.5286) -> (-29.5395, 33.9371) centre (-0.3, 19.45) ccw
  spline S1 degree 3 poles (-28.303, 31.0492) (-28.5681, 31.159) (-28.8568, 31.3466) (-29.2595, 31.7355) (-29.4492, 32.0024) (-29.6648, 32.4884) (-29.734, 32.7911) (-29.7424, 33.2981) (-29.6876, 33.5909) (-29.5926, 33.8202) (-29.5767, 33.8587) (-29.559, 33.8979) (-29.5395, 33.9371) knots -0.320047 -0.320047 -0.320047 -0.320047 -0.233978 -0.233978 -0.152103 -0.152103 -0.074471 -0.074471 0 0 0 0.012509 0.012509 0.012509 0.012509
  spline S2 degree 3 poles (-21.8612, 43.9437) (-21.8284, 43.9726) (-21.7951, 43.9998) (-21.7621, 44.0252) (-21.5651, 44.1763) (-21.2965, 44.305) (-20.8046, 44.4281) (-20.4943, 44.4397) (-19.9691, 44.3572) (-19.6621, 44.243) (-19.1823, 43.9547) (-18.9264, 43.7244) (-18.7517, 43.4968) knots -0.012509 -0.012509 -0.012509 -0.012509 0 0 0 0.074471 0.074471 0.152103 0.152103 0.233978 0.233978 0.320047 0.320047 0.320047 0.320047
  arc A2 (-21.8612, 43.9437) -> (-24.7937, 41.0112) centre (-0.3, 19.45) ccw
  spline S3 degree 3 poles (-24.3468, 37.9017) (-24.5744, 38.0764) (-24.8047, 38.3323) (-25.093, 38.8121) (-25.2072, 39.1191) (-25.2897, 39.6443) (-25.2781, 39.9546) (-25.155, 40.4465) (-25.0263, 40.7151) (-24.8752, 40.9121) (-24.8498, 40.9451) (-24.8226, 40.9784) (-24.7937, 41.0112) knots -0.320047 -0.320047 -0.320047 -0.320047 -0.233978 -0.233978 -0.152103 -0.152103 -0.074471 -0.074471 0 0 0 0.012509 0.012509 0.012509 0.012509
  spline S4 degree 3 poles (-14.7871, 48.6895) (-14.7479, 48.709) (-14.7087, 48.7267) (-14.6702, 48.7426) (-14.4409, 48.8376) (-14.1481, 48.8924) (-13.6411, 48.884) (-13.3384, 48.8148) (-12.8524, 48.5992) (-12.5855, 48.4095) (-12.1966, 48.0068) (-12.009, 47.7181) (-11.8992, 47.453) knots -0.012509 -0.012509 -0.012509 -0.012509 0 0 0 0.074471 0.074471 0.152103 0.152103 0.233978 0.233978 0.320047 0.320047 0.320047 0.320047
  arc A3 (-14.7871, 48.6895) -> (-18.3786, 46.616) centre (-0.3, 19.45) ccw
  spline S5 degree 3 poles (-18.7517, 43.4968) (-18.9264, 43.7244) (-19.0826, 44.0311) (-19.2369, 44.5693) (-19.2678, 44.8953) (-19.2115, 45.424) (-19.12, 45.7208) (-18.8738, 46.164) (-18.68, 46.3902) (-18.4831, 46.5413) (-18.45, 46.5667) (-18.4151, 46.5917) (-18.3786, 46.616) knots -0.320047 -0.320047 -0.320047 -0.320047 -0.233978 -0.233978 -0.152103 -0.152103 -0.074471 -0.074471 0 0 0 0.012509 0.012509 0.012509 0.012509
  spline S6 degree 3 poles (-6.7257, 51.4428) (-6.6828, 51.4514) (-6.6404, 51.4584) (-6.5991, 51.4638) (-6.353, 51.4962) (-6.056, 51.4733) (-5.5685, 51.334) (-5.294, 51.1888) (-4.8803, 50.8548) (-4.6716, 50.6024) (-4.4002, 50.1128) (-4.2937, 49.7854) (-4.2563, 49.501) knots -0.012509 -0.012509 -0.012509 -0.012509 0 0 0 0.074471 0.074471 0.152103 0.152103 0.233978 0.233978 0.320047 0.320047 0.320047 0.320047
  arc A4 (-6.7257, 51.4428) -> (-10.7315, 50.3694) centre (-0.3, 19.45) ccw
  spline S7 degree 3 poles (-11.8992, 47.453) (-12.009, 47.7181) (-12.0806, 48.0549) (-12.0903, 48.6146) (-12.0357, 48.9375) (-11.8445, 49.4336) (-11.6794, 49.6966) (-11.3269, 50.061) (-11.0811, 50.2293) (-10.8517, 50.3243) (-10.8132, 50.3403) (-10.773, 50.3554) (-10.7315, 50.3694) knots -0.320047 -0.320047 -0.320047 -0.320047 -0.233978 -0.233978 -0.152103 -0.152103 -0.074471 -0.074471 0 0 0 0.012509 0.012509 0.012509 0.012509
  spline S8 degree 3 poles (1.7736, 52.0157) (1.8172, 52.013) (1.86, 52.0087) (1.9013, 52.0033) (2.1475, 51.9709) (2.4284, 51.8719) (2.8632, 51.6112) (3.0908, 51.3999) (3.4039, 50.9702) (3.5402, 50.6724) (3.6757, 50.1292) (3.6937, 49.7854) (3.6563, 49.501) knots -0.012509 -0.012509 -0.012509 -0.012509 0 0 0 0.074471 0.074471 0.152103 0.152103 0.233978 0.233978 0.320047 0.320047 0.320047 0.320047
  arc A5 (1.7736, 52.0157) -> (-2.3736, 52.0157) centre (-0.3, 19.45) ccw
  spline S9 degree 3 poles (-4.2563, 49.501) (-4.2937, 49.7854) (-4.2757, 50.1292) (-4.1402, 50.6724) (-4.0039, 50.9702) (-3.6908, 51.3999) (-3.4632, 51.6112) (-3.0284, 51.8719) (-2.7475, 51.9709) (-2.5013, 52.0033) (-2.46, 52.0087) (-2.4172, 52.013) (-2.3736, 52.0157) knots -0.320047 -0.320047 -0.320047 -0.320047 -0.233978 -0.233978 -0.152103 -0.152103 -0.074471 -0.074471 0 0 0 0.012509 0.012509 0.012509 0.012509
  spline S10 degree 3 poles (10.1315, 50.3694) (10.173, 50.3554) (10.2132, 50.3403) (10.2517, 50.3243) (10.4811, 50.2293) (10.7269, 50.061) (11.0794, 49.6966) (11.2445, 49.4336) (11.4357, 48.9375) (11.4903, 48.6146) (11.4806, 48.0549) (11.409, 47.7181) (11.2992, 47.453) knots -0.012509 -0.012509 -0.012509 -0.012509 0 0 0 0.074471 0.074471 0.152103 0.152103 0.233978 0.233978 0.320047 0.320047 0.320047 0.320047
  arc A6 (10.1315, 50.3694) -> (6.1257, 51.4428) centre (-0.3, 19.45) ccw
  spline S11 degree 3 poles (3.6563, 49.501) (3.6937, 49.7854) (3.8002, 50.1128) (4.0716, 50.6024) (4.2803, 50.8548) (4.694, 51.1888) (4.9685, 51.334) (5.456, 51.4733) (5.753, 51.4962) (5.9991, 51.4638) (6.0404, 51.4584) (6.0828, 51.4514) (6.1257, 51.4428) knots -0.320047 -0.320047 -0.320047 -0.320047 -0.233978 -0.233978 -0.152103 -0.152103 -0.074471 -0.074471 0 0 0 0.012509 0.012509 0.012509 0.012509
  spline S12 degree 3 poles (17.7786, 46.616) (17.8151, 46.5917) (17.85, 46.5667) (17.8831, 46.5413) (18.08, 46.3902) (18.2738, 46.164) (18.52, 45.7208) (18.6115, 45.424) (18.6678, 44.8953) (18.6369, 44.5693) (18.4826, 44.0311) (18.3264, 43.7244) (18.1517, 43.4968) knots -0.012509 -0.012509 -0.012509 -0.012509 0 0 0 0.074471 0.074471 0.152103 0.152103 0.233978 0.233978 0.320047 0.320047 0.320047 0.320047
  arc A7 (17.7786, 46.616) -> (14.1871, 48.6895) centre (-0.3, 19.45) ccw
  spline S13 degree 3 poles (11.2992, 47.453) (11.409, 47.7181) (11.5966, 48.0068) (11.9855, 48.4095) (12.2524, 48.5992) (12.7384, 48.8148) (13.0411, 48.884) (13.5481, 48.8924) (13.8409, 48.8376) (14.0702, 48.7426) (14.1087, 48.7267) (14.1479, 48.709) (14.1871, 48.6895) knots -0.320047 -0.320047 -0.320047 -0.320047 -0.233978 -0.233978 -0.152103 -0.152103 -0.074471 -0.074471 0 0 0 0.012509 0.012509 0.012509 0.012509
  spline S14 degree 3 poles (24.1937, 41.0112) (24.2226, 40.9784) (24.2498, 40.9451) (24.2752, 40.9121) (24.4263, 40.7151) (24.555, 40.4465) (24.6781, 39.9546) (24.6897, 39.6443) (24.6072, 39.1191) (24.493, 38.8121) (24.2047, 38.3323) (23.9744, 38.0764) (23.7468, 37.9017) knots -0.012509 -0.012509 -0.012509 -0.012509 0 0 0 0.074471 0.074471 0.152103 0.152103 0.233978 0.233978 0.320047 0.320047 0.320047 0.320047
  arc A8 (24.1937, 41.0112) -> (21.2612, 43.9437) centre (-0.3, 19.45) ccw
  spline S15 degree 3 poles (18.1517, 43.4968) (18.3264, 43.7244) (18.5823, 43.9547) (19.0621, 44.243) (19.3691, 44.3572) (19.8943, 44.4397) (20.2046, 44.4281) (20.6965, 44.305) (20.9651, 44.1763) (21.1621, 44.0252) (21.1951, 43.9998) (21.2284, 43.9726) (21.2612, 43.9437) knots -0.320047 -0.320047 -0.320047 -0.320047 -0.233978 -0.233978 -0.152103 -0.152103 -0.074471 -0.074471 0 0 0 0.012509 0.012509 0.012509 0.012509
  spline S16 degree 3 poles (28.9395, 33.9371) (28.959, 33.8979) (28.9767, 33.8587) (28.9926, 33.8202) (29.0876, 33.5909) (29.1424, 33.2981) (29.134, 32.7911) (29.0648, 32.4884) (28.8492, 32.0024) (28.6595, 31.7355) (28.2568, 31.3466) (27.9681, 31.159) (27.703, 31.0492) knots -0.012509 -0.012509 -0.012509 -0.012509 0 0 0 0.074471 0.074471 0.152103 0.152103 0.233978 0.233978 0.320047 0.320047 0.320047 0.320047
  arc A9 (28.9395, 33.9371) -> (26.866, 37.5286) centre (-0.3, 19.45) ccw
  spline S17 degree 3 poles (23.7468, 37.9017) (23.9744, 38.0764) (24.2811, 38.2326) (24.8193, 38.3869) (25.1453, 38.4178) (25.674, 38.3615) (25.9708, 38.27) (26.414, 38.0238) (26.6402, 37.83) (26.7913, 37.6331) (26.8167, 37.6) (26.8417, 37.5651) (26.866, 37.5286) knots -0.320047 -0.320047 -0.320047 -0.320047 -0.233978 -0.233978 -0.152103 -0.152103 -0.074471 -0.074471 0 0 0 0.012509 0.012509 0.012509 0.012509
  spline S18 degree 3 poles (31.6928, 25.8757) (31.7014, 25.8328) (31.7084, 25.7904) (31.7138, 25.7491) (31.7462, 25.503) (31.7233, 25.206) (31.584, 24.7185) (31.4388, 24.444) (31.1048, 24.0303) (30.8524, 23.8216) (30.3628, 23.5502) (30.0354, 23.4437) (29.751, 23.4063) knots -0.012509 -0.012509 -0.012509 -0.012509 0 0 0 0.074471 0.074471 0.152103 0.152103 0.233978 0.233978 0.320047 0.320047 0.320047 0.320047
  arc A10 (31.6928, 25.8757) -> (30.6194, 29.8815) centre (-0.3, 19.45) ccw
  spline S19 degree 3 poles (27.703, 31.0492) (27.9681, 31.159) (28.3049, 31.2306) (28.8646, 31.2403) (29.1875, 31.1857) (29.6836, 30.9945) (29.9466, 30.8294) (30.311, 30.4769) (30.4793, 30.2311) (30.5743, 30.0017) (30.5903, 29.9632) (30.6054, 29.923) (30.6194, 29.8815) knots -0.320047 -0.320047 -0.320047 -0.320047 -0.233978 -0.233978 -0.152103 -0.152103 -0.074471 -0.074471 0 0 0 0.012509 0.012509 0.012509 0.012509
  spline S20 degree 3 poles (32.2657, 17.3764) (32.263, 17.3328) (32.2587, 17.29) (32.2533, 17.2487) (32.2209, 17.0025) (32.1219, 16.7216) (31.8612, 16.2868) (31.6499, 16.0592) (31.2202, 15.7461) (30.9224, 15.6098) (30.3792, 15.4743) (30.0354, 15.4563) (29.751, 15.4937) knots -0.012509 -0.012509 -0.012509 -0.012509 0 0 0 0.074471 0.074471 0.152103 0.152103 0.233978 0.233978 0.320047 0.320047 0.320047 0.320047
  arc A11 (32.2657, 17.3764) -> (32.2657, 21.5236) centre (-0.3, 19.45) ccw
  spline S21 degree 3 poles (29.751, 23.4063) (30.0354, 23.4437) (30.3792, 23.4257) (30.9224, 23.2902) (31.2202, 23.1539) (31.6499, 22.8408) (31.8612, 22.6132) (32.1219, 22.1784) (32.2209, 21.8975) (32.2533, 21.6513) (32.2587, 21.61) (32.263, 21.5672) (32.2657, 21.5236) knots -0.320047 -0.320047 -0.320047 -0.320047 -0.233978 -0.233978 -0.152103 -0.152103 -0.074471 -0.074471 0 0 0 0.012509 0.012509 0.012509 0.012509
  spline S22 degree 3 poles (30.6194, 9.0185) (30.6054, 8.977) (30.5903, 8.9368) (30.5743, 8.8983) (30.4793, 8.6689) (30.311, 8.4231) (29.9466, 8.0706) (29.6836, 7.9055) (29.1875, 7.7143) (28.8646, 7.6597) (28.3049, 7.6694) (27.9681, 7.741) (27.703, 7.8508) knots -0.012509 -0.012509 -0.012509 -0.012509 0 0 0 0.074471 0.074471 0.152103 0.152103 0.233978 0.233978 0.320047 0.320047 0.320047 0.320047
  arc A12 (30.6194, 9.0185) -> (31.6928, 13.0243) centre (-0.3, 19.45) ccw
  spline S23 degree 3 poles (29.751, 15.4937) (30.0354, 15.4563) (30.3628, 15.3498) (30.8524, 15.0784) (31.1048, 14.8697) (31.4388, 14.456) (31.584, 14.1815) (31.7233, 13.694) (31.7462, 13.397) (31.7138, 13.1509) (31.7084, 13.1096) (31.7014, 13.0672) (31.6928, 13.0243) knots -0.320047 -0.320047 -0.320047 -0.320047 -0.233978 -0.233978 -0.152103 -0.152103 -0.074471 -0.074471 0 0 0 0.012509 0.012509 0.012509 0.012509
  spline S24 degree 3 poles (26.866, 1.3714) (26.8417, 1.3349) (26.8167, 1.3) (26.7913, 1.2669) (26.6402, 1.07) (26.414, 0.8762) (25.9708, 0.63) (25.674, 0.5385) (25.1453, 0.4822) (24.8193, 0.5131) (24.2811, 0.6674) (23.9744, 0.8236) (23.7468, 0.9983) knots -0.012509 -0.012509 -0.012509 -0.012509 0 0 0 0.074471 0.074471 0.152103 0.152103 0.233978 0.233978 0.320047 0.320047 0.320047 0.320047
  arc A13 (26.866, 1.3714) -> (28.9395, 4.9629) centre (-0.3, 19.45) ccw
  spline S25 degree 3 poles (27.703, 7.8508) (27.9681, 7.741) (28.2568, 7.5534) (28.6595, 7.1645) (28.8492, 6.8976) (29.0648, 6.4116) (29.134, 6.1089) (29.1424, 5.6019) (29.0876, 5.3091) (28.9926, 5.0798) (28.9767, 5.0413) (28.959, 5.0021) (28.9395, 4.9629) knots -0.320047 -0.320047 -0.320047 -0.320047 -0.233978 -0.233978 -0.152103 -0.152103 -0.074471 -0.074471 0 0 0 0.012509 0.012509 0.012509 0.012509
  spline S26 degree 3 poles (21.2612, -5.0437) (21.2284, -5.0726) (21.1951, -5.0998) (21.1621, -5.1252) (20.9651, -5.2763) (20.6965, -5.405) (20.2046, -5.5281) (19.8943, -5.5397) (19.3691, -5.4572) (19.0621, -5.343) (18.5823, -5.0547) (18.3264, -4.8244) (18.1517, -4.5968) knots -0.012509 -0.012509 -0.012509 -0.012509 0 0 0 0.074471 0.074471 0.152103 0.152103 0.233978 0.233978 0.320047 0.320047 0.320047 0.320047
  arc A14 (21.2612, -5.0437) -> (24.1937, -2.1112) centre (-0.3, 19.45) ccw
  spline S27 degree 3 poles (23.7468, 0.9983) (23.9744, 0.8236) (24.2047, 0.5677) (24.493, 0.0879) (24.6072, -0.2191) (24.6897, -0.7443) (24.6781, -1.0546) (24.555, -1.5465) (24.4263, -1.8151) (24.2752, -2.0121) (24.2498, -2.0451) (24.2226, -2.0784) (24.1937, -2.1112) knots -0.320047 -0.320047 -0.320047 -0.320047 -0.233978 -0.233978 -0.152103 -0.152103 -0.074471 -0.074471 0 0 0 0.012509 0.012509 0.012509 0.012509
  spline S28 degree 3 poles (14.1871, -9.7895) (14.1479, -9.809) (14.1087, -9.8267) (14.0702, -9.8426) (13.8409, -9.9376) (13.5481, -9.9924) (13.0411, -9.984) (12.7384, -9.9148) (12.2524, -9.6992) (11.9855, -9.5095) (11.5966, -9.1068) (11.409, -8.8181) (11.2992, -8.553) knots -0.012509 -0.012509 -0.012509 -0.012509 0 0 0 0.074471 0.074471 0.152103 0.152103 0.233978 0.233978 0.320047 0.320047 0.320047 0.320047
  arc A15 (14.1871, -9.7895) -> (17.7786, -7.716) centre (-0.3, 19.45) ccw
  spline S29 degree 3 poles (18.1517, -4.5968) (18.3264, -4.8244) (18.4826, -5.1311) (18.6369, -5.6693) (18.6678, -5.9953) (18.6115, -6.524) (18.52, -6.8208) (18.2738, -7.264) (18.08, -7.4902) (17.8831, -7.6413) (17.85, -7.6667) (17.8151, -7.6917) (17.7786, -7.716) knots -0.320047 -0.320047 -0.320047 -0.320047 -0.233978 -0.233978 -0.152103 -0.152103 -0.074471 -0.074471 0 0 0 0.012509 0.012509 0.012509 0.012509
  spline S30 degree 3 poles (6.1257, -12.5428) (6.0828, -12.5514) (6.0404, -12.5584) (5.9991, -12.5638) (5.753, -12.5962) (5.456, -12.5733) (4.9685, -12.434) (4.694, -12.2888) (4.2803, -11.9548) (4.0716, -11.7024) (3.8002, -11.2128) (3.6937, -10.8854) (3.6563, -10.601) knots -0.012509 -0.012509 -0.012509 -0.012509 0 0 0 0.074471 0.074471 0.152103 0.152103 0.233978 0.233978 0.320047 0.320047 0.320047 0.320047
  arc A16 (6.1257, -12.5428) -> (10.1315, -11.4694) centre (-0.3, 19.45) ccw
  spline S31 degree 3 poles (11.2992, -8.553) (11.409, -8.8181) (11.4806, -9.1549) (11.4903, -9.7146) (11.4357, -10.0375) (11.2445, -10.5336) (11.0794, -10.7966) (10.7269, -11.161) (10.4811, -11.3293) (10.2517, -11.4243) (10.2132, -11.4403) (10.173, -11.4554) (10.1315, -11.4694) knots -0.320047 -0.320047 -0.320047 -0.320047 -0.233978 -0.233978 -0.152103 -0.152103 -0.074471 -0.074471 0 0 0 0.012509 0.012509 0.012509 0.012509
  spline S32 degree 3 poles (-2.3736, -13.1157) (-2.4172, -13.113) (-2.46, -13.1087) (-2.5013, -13.1033) (-2.7475, -13.0709) (-3.0284, -12.9719) (-3.4632, -12.7112) (-3.6908, -12.4999) (-4.0039, -12.0702) (-4.1402, -11.7724) (-4.2757, -11.2292) (-4.2937, -10.8854) (-4.2563, -10.601) knots -0.012509 -0.012509 -0.012509 -0.012509 0 0 0 0.074471 0.074471 0.152103 0.152103 0.233978 0.233978 0.320047 0.320047 0.320047 0.320047
  arc A17 (-2.3736, -13.1157) -> (1.7736, -13.1157) centre (-0.3, 19.45) ccw
  spline S33 degree 3 poles (3.6563, -10.601) (3.6937, -10.8854) (3.6757, -11.2292) (3.5402, -11.7724) (3.4039, -12.0702) (3.0908, -12.4999) (2.8632, -12.7112) (2.4284, -12.9719) (2.1475, -13.0709) (1.9013, -13.1033) (1.86, -13.1087) (1.8172, -13.113) (1.7736, -13.1157) knots -0.320047 -0.320047 -0.320047 -0.320047 -0.233978 -0.233978 -0.152103 -0.152103 -0.074471 -0.074471 0 0 0 0.012509 0.012509 0.012509 0.012509
  spline S34 degree 3 poles (-10.7315, -11.4694) (-10.773, -11.4554) (-10.8132, -11.4403) (-10.8517, -11.4243) (-11.0811, -11.3293) (-11.3269, -11.161) (-11.6794, -10.7966) (-11.8445, -10.5336) (-12.0357, -10.0375) (-12.0903, -9.7146) (-12.0806, -9.1549) (-12.009, -8.8181) (-11.8992, -8.553) knots -0.012509 -0.012509 -0.012509 -0.012509 0 0 0 0.074471 0.074471 0.152103 0.152103 0.233978 0.233978 0.320047 0.320047 0.320047 0.320047
  arc A18 (-10.7315, -11.4694) -> (-6.7257, -12.5428) centre (-0.3, 19.45) ccw
  spline S35 degree 3 poles (-4.2563, -10.601) (-4.2937, -10.8854) (-4.4002, -11.2128) (-4.6716, -11.7024) (-4.8803, -11.9548) (-5.294, -12.2888) (-5.5685, -12.434) (-6.056, -12.5733) (-6.353, -12.5962) (-6.5991, -12.5638) (-6.6404, -12.5584) (-6.6828, -12.5514) (-6.7257, -12.5428) knots -0.320047 -0.320047 -0.320047 -0.320047 -0.233978 -0.233978 -0.152103 -0.152103 -0.074471 -0.074471 0 0 0 0.012509 0.012509 0.012509 0.012509
  spline S36 degree 3 poles (-18.3786, -7.716) (-18.4151, -7.6917) (-18.45, -7.6667) (-18.4831, -7.6413) (-18.68, -7.4902) (-18.8738, -7.264) (-19.12, -6.8208) (-19.2115, -6.524) (-19.2678, -5.9953) (-19.2369, -5.6693) (-19.0826, -5.1311) (-18.9264, -4.8244) (-18.7517, -4.5968) knots -0.012509 -0.012509 -0.012509 -0.012509 0 0 0 0.074471 0.074471 0.152103 0.152103 0.233978 0.233978 0.320047 0.320047 0.320047 0.320047
  arc A19 (-18.3786, -7.716) -> (-14.7871, -9.7895) centre (-0.3, 19.45) ccw
  spline S37 degree 3 poles (-11.8992, -8.553) (-12.009, -8.8181) (-12.1966, -9.1068) (-12.5855, -9.5095) (-12.8524, -9.6992) (-13.3384, -9.9148) (-13.6411, -9.984) (-14.1481, -9.9924) (-14.4409, -9.9376) (-14.6702, -9.8426) (-14.7087, -9.8267) (-14.7479, -9.809) (-14.7871, -9.7895) knots -0.320047 -0.320047 -0.320047 -0.320047 -0.233978 -0.233978 -0.152103 -0.152103 -0.074471 -0.074471 0 0 0 0.012509 0.012509 0.012509 0.012509
  spline S38 degree 3 poles (-24.7937, -2.1112) (-24.8226, -2.0784) (-24.8498, -2.0451) (-24.8752, -2.0121) (-25.0263, -1.8151) (-25.155, -1.5465) (-25.2781, -1.0546) (-25.2897, -0.7443) (-25.2072, -0.2191) (-25.093, 0.0879) (-24.8047, 0.5677) (-24.5744, 0.8236) (-24.3468, 0.9983) knots -0.012509 -0.012509 -0.012509 -0.012509 0 0 0 0.074471 0.074471 0.152103 0.152103 0.233978 0.233978 0.320047 0.320047 0.320047 0.320047
  arc A20 (-24.7937, -2.1112) -> (-21.8612, -5.0437) centre (-0.3, 19.45) ccw
  spline S39 degree 3 poles (-18.7517, -4.5968) (-18.9264, -4.8244) (-19.1823, -5.0547) (-19.6621, -5.343) (-19.9691, -5.4572) (-20.4943, -5.5397) (-20.8046, -5.5281) (-21.2965, -5.405) (-21.5651, -5.2763) (-21.7621, -5.1252) (-21.7951, -5.0998) (-21.8284, -5.0726) (-21.8612, -5.0437) knots -0.320047 -0.320047 -0.320047 -0.320047 -0.233978 -0.233978 -0.152103 -0.152103 -0.074471 -0.074471 0 0 0 0.012509 0.012509 0.012509 0.012509
  spline S40 degree 3 poles (-29.5395, 4.9629) (-29.559, 5.0021) (-29.5767, 5.0413) (-29.5926, 5.0798) (-29.6876, 5.3091) (-29.7424, 5.6019) (-29.734, 6.1089) (-29.6648, 6.4116) (-29.4492, 6.8976) (-29.2595, 7.1645) (-28.8568, 7.5534) (-28.5681, 7.741) (-28.303, 7.8508) knots -0.012509 -0.012509 -0.012509 -0.012509 0 0 0 0.074471 0.074471 0.152103 0.152103 0.233978 0.233978 0.320047 0.320047 0.320047 0.320047
  arc A21 (-29.5395, 4.9629) -> (-27.466, 1.3714) centre (-0.3, 19.45) ccw